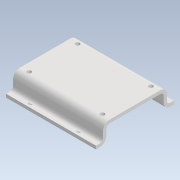
# Autodesk Inventor part: BaseMotor
Saved by Autodesk Inventor 2021 (Build 250183000, 183)
## iProperties
Created: 2021-08-18
Part Number: BaseMotor
Material: Generic
Document SubType Name: Sheet Metal
Designer: Santiago Suárez
Density: 1 g/cm^3
Sheet Metal Rule: Default_mm
Appearance: Default
Flat Pattern Width: 26 cm
Flat Pattern Length: 32.3954 cm
Flat Pattern Area: 842.28 cm^2
Sheet Metal Width: 260,000 mm
Sheet Metal Length: 323,954 mm
Sheet Metal Area: 84228,034 mm^2
Author: Santiago Suárez
Autodesk Inventor part; units mm, degrees
ref_plane "YZ Plane" through (0, 0, 0) normal (1, 0, 0) x (0, 1, 0)
ref_plane "XZ Plane" through (0, 0, 0) normal (0, 1, 0) x (-1, 0, 0)
ref_plane "XY Plane" through (0, 0, 0) normal (0, 0, 1) x (1, 0, 0)
sketch "Sketch1" plane through (0, 0, 0) normal (0, 1, 0) x (-1, 0, 0)
  line L0 (130, 100) -> (-130, 100)
  line L1 (-130, 100) -> (-130, -100)
  line L2 (-130, -100) -> (130, -100)
  line L3 (130, -100) -> (130, 100)
  point P0 (0, 0)
  dimension "d0" = 260
  dimension "d1" = 200
  dimension "d2" = 100
  dimension "d29" = 130
  measures "d0" distance of L0.start L0.end
  measures "d1" distance of L2.end L0.start
  measures "d2" distance from line of L0 point (0, 0)
  measures "d29" distance from line of L3 point (0, 0)
extrude "Plate1" add sketch "Sketch1" along normal blind 9.5
sketch "Sketch2" plane through (130, 9.5, 90.5) normal (0, 0, 1) x (1, 0, 0)
  line L0 (-260, 0) -> (0, 0)
  line L1 (0, 0) -> (0, 55)
  line L2 (0, 55) -> (-260, 55)
  line L3 (-260, 55) -> (-260, 0)
  constraints: 6 end point, 1 horizontal, 1 perpendicular, 1 vertical
edge flange "Flange1" height 55 angle 90 thickness 9.5 bend radius 9.5 thickness toward (0, 0, 1) relief straight relief width 9.5 relief depth 4.75 edges at (0, 9.5, 100) wall of the first edge with corners at (-130, 9.5, 90.5) (130, 9.5, 90.5) (130, -45.5, 90.5) (-130, -45.5, 90.5)
bend "Bend1"
corner "Corner1"
sketch "Sketch3" plane through (-130, 9.5, -90.5) normal (0, 0, -1) x (-1, 0, 0)
  line L0 (-260, 0) -> (0, 0)
  line L1 (0, 0) -> (0, 55)
  line L2 (0, 55) -> (-260, 55)
  line L3 (-260, 55) -> (-260, 0)
  constraints: 6 end point, 1 horizontal, 1 perpendicular, 1 vertical
edge flange "Flange2" height 55 angle 90 thickness 9.5 bend radius 9.5 thickness toward (0, 0, -1) relief straight relief width 9.5 relief depth 4.75 edges at (0, 9.5, -100) wall of the first edge with corners at (130, 9.5, -90.5) (-130, 9.5, -90.5) (-130, -45.5, -90.5) (130, -45.5, -90.5)
bend "Bend2"
corner "Corner2"
sketch "Sketch4" plane through (0, 9.5, 0) normal (0, 1, 0) x (1, 0, 0)
  line L0 (-106, -70) -> (106, -70)
  line L1 (106, -70) -> (106, 70)
  line L2 (106, 70) -> (-106, 70)
  line L3 (-106, 70) -> (-106, -70)
  line L4 (-130, -81) -> (-130, 81) projected
  point P0 (0, 0)
  dimension "d24" = 140
  dimension "d25" = 212
  dimension "d27" = 70
  dimension "d28" = 106
  constraints: 8 end point, 4 coincident, 2 parallel, 1 horizontal, 1 perpendicular
  measures "d24" distance of L2.end L0.start
  measures "d25" distance of L0.start L0.end
  measures "d27" distance from line of point (0, 0) L0
  measures "d28" distance from line of point (0, 0) L3
hole "Hole1" at (-106, 9.5, 70) at (-106, 9.5, -70) at (106, 9.5, 70) at (106, 9.5, -70) direction (0, -1, 0) diameter 12 depth 9.5
sketch "Sketch5" plane through (130, -36, -90.5) normal (0, -1, 0) x (1, 0, 0)
  line L0 (-260, 0) -> (0, 0)
  line L1 (0, 0) -> (0, 40)
  line L2 (0, 40) -> (-260, 40)
  line L3 (-260, 40) -> (-260, 0)
  constraints: 6 end point, 1 horizontal, 1 perpendicular, 1 vertical
edge flange "Flange3" height 40 angle 90 thickness 9.5 bend radius 9.5 thickness toward (0, -1, 0) relief straight relief width 9.5 relief depth 4.75 edges at (0, -45.5, -90.5) wall of the first edge with corners at (-130, -36, -90.5) (130, -36, -90.5) (130, -36, -130.5) (-130, -36, -130.5)
bend "Bend3"
corner "Corner3"
sketch "Sketch6" plane through (-130, -36, 90.5) normal (0, -1, 0) x (1, 0, 0)
  line L0 (260, 0) -> (0, 0)
  line L1 (0, 0) -> (0, -40)
  line L2 (0, -40) -> (260, -40)
  line L3 (260, -40) -> (260, 0)
  constraints: 6 end point, 1 horizontal, 1 perpendicular, 1 vertical
edge flange "Flange4" height 40 angle 90 thickness 9.5 bend radius 9.5 thickness toward (0, -1, 0) relief straight relief width 9.5 relief depth 4.75 edges at (0, -45.5, 90.5) wall of the first edge with corners at (130, -36, 90.5) (-130, -36, 90.5) (-130, -36, 130.5) (130, -36, 130.5)
bend "Bend4"
corner "Corner4"
sketch "Sketch7" plane through (-130, -36, 130.5) normal (0, 1, 0) x (1, 0, 0)
  line L0 (0, 21) -> (0, 0) projected
  line L1 (260, 0) -> (0, 0) projected
  line L2 (60, 0) -> (60, 24)
  line L3 (200, 0) -> (200, 24)
  line L4 (260, 21) -> (260, 0) projected
  point P0 (130, 130.5)
  point P1 (60, 10)
  point P2 (200, 10)
  dimension "d57" = 60
  dimension "d58" = 60
  dimension "d66" = 10
  dimension "d67" = 10
  constraints: 4 end point, 4 point on line, 1 vertical
  measures "d57" distance between parallel lines of L3 L4
  measures "d58" distance between parallel lines of L2 L0
  measures "d66" distance from line of L1 point (60, 10)
  measures "d67" distance from line of L1 point (200, 10)
hole "Hole2" at (-70, -36, 120.5) at (70, -36, 120.5) direction (0, -1, 0) diameter 12 depth 9.5
mirror "Mirror1" about plane through (0, 0, 0) normal (0, 0, 1) of "Hole2"
equation "\"d28\" = 0.5 * d25"
equation "\"d35\" = Thickness"
equation "\"d64\" = Thickness"
equation "\"d3\" = Thickness"
equation "\"d4\" = BendReliefWidth"
equation "\"d5\" = BendReliefDepth"
equation "\"d6\" = MinimumRemnant"
equation "\"d7\" = TransitionRadius"
equation "\"d10\" = BendRadius"
equation "\"d11\" = CornerReliefSize"
equation "\"d12\" = GapSize"
equation "\"d13\" = JacobiRadiusSize"
equation "\"d14\" = BendReliefWidth"
equation "\"d15\" = BendReliefDepth"
equation "\"d16\" = MinimumRemnant"
equation "\"d17\" = TransitionRadius"
equation "\"d20\" = BendRadius"
equation "\"d21\" = CornerReliefSize"
equation "\"d22\" = GapSize"
equation "\"d23\" = JacobiRadiusSize"
equation "\"d37\" = BendReliefWidth"
equation "\"d38\" = BendReliefDepth"
equation "\"d39\" = MinimumRemnant"
equation "\"d40\" = TransitionRadius"
equation "\"d43\" = BendRadius"
equation "\"d44\" = CornerReliefSize"
equation "\"d45\" = GapSize"
equation "\"d46\" = JacobiRadiusSize"
equation "\"d47\" = BendReliefWidth"
equation "\"d48\" = BendReliefDepth"
equation "\"d49\" = MinimumRemnant"
equation "\"d50\" = TransitionRadius"
equation "\"d53\" = BendRadius"
equation "\"d54\" = CornerReliefSize"
equation "\"d55\" = GapSize"
equation "\"d56\" = JacobiRadiusSize"
equation "\"d2\" = 0.5 * d1"
equation "\"d29\" = 0.5 * d0"
equation "\"BendRadius\" = Thickness"
equation "\"BendReliefWidth\" = Thickness"
equation "\"BendReliefDepth\" = 0.5 * Thickness"
equation "\"CornerReliefSize\" = 4 * Thickness"
equation "\"MinimumRemnant\" = 2 * Thickness"
equation "\"TransitionRadius\" = BendRadius"
equation "\"JacobiRadiusSize\" = BendRadius"
equation "\"GapSize\" = Thickness"
equation "\"Thickness\" = 9.5"
body "Solid1"
